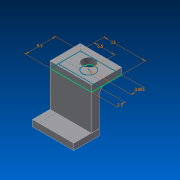
# Autodesk Inventor part: ethernet bracket support
Saved by Autodesk Inventor 2015 (Build 190159000, 159)
## iProperties
Created: 2017-03-16
Part Number: ethernet bracket support
Material: Generic
Document SubType Name: Modeling
Designer: ZigZagJoe
Density: 1 g/cm^3
Appearance: Default
Author: ZigZagJoe
Autodesk Inventor part; units mm, degrees
ref_plane "YZ Plane" through (0, 0, 0) normal (1, 0, 0) x (0, 1, 0)
ref_plane "XZ Plane" through (0, 0, 0) normal (0, 1, 0) x (-1, 0, 0)
ref_plane "XY Plane" through (0, 0, 0) normal (0, 0, 1) x (1, 0, 0)
sketch "Sketch1" plane through (0, 0, 0) normal (0, 0, 1) x (1, 0, 0)
  line L0 (-5.976, 1.765) -> (7.024, 1.765)
  line L1 (7.024, 1.765) -> (7.024, -7.735)
  line L2 (7.024, -7.735) -> (-5.976, -7.735)
  line L3 (-5.976, -7.735) -> (-5.976, 1.765)
  line L4 (-5.976, -7.735) -> (7.024, -7.735)
  line L5 (7.024, -7.735) -> (7.024, -5.235)
  line L6 (7.024, -5.235) -> (-5.976, -5.235)
  line L7 (-5.976, -5.235) -> (-5.976, -7.735)
  circle A0 centre (0.524, -2.0964) radius 2
  point P0 (0, 0)
  dimension "d0" = 9.5
  dimension "d1" = 13
  dimension "d2" = 2.5
  dimension "d3" = 4
  dimension "d4" = 6.5
  dimension "d5" = 3.8614
  constraints: 16 end point, 4 parallel, 2 horizontal, 2 perpendicular, 1 centre point, 1 point on line
  measures "d0" distance of L2.end L0.start
  measures "d1" distance of L0.start L0.end
  measures "d2" distance between parallel lines of L2 L6
  measures "d3" diameter of A0
  measures "d4" distance from line of L3 A0.centre
  measures "d5" distance from line of L0 A0.centre
extrude "Extrusion1" add sketch "Sketch1" along normal blind 2
extrude "Extrusion2" add sketch "Sketch1" against normal blind 11.2 contours L6 L1 L2 L3
sketch "Sketch2" plane through (0, 0, -11.2) normal (0, 0, -1) x (-1, 0, 0)
  line L0 (-6.988, -5.235) -> (5.976, -5.235)
  line L1 (5.976, -5.235) -> (5.976, -13.235)
  line L2 (5.976, -13.235) -> (-6.988, -13.235)
  line L3 (-6.988, -13.235) -> (-6.988, -5.235)
  line L4 (5.976, -7.735) -> (5.976, -5.235) projected
  line L5 (5.976, -5.235) -> (-7.024, -5.235) projected
  point P0 (0, 0)
  dimension "d10" = 0
  dimension "d11" = 8
  dimension "d12" = 0
  constraints: 8 end point, 2 parallel, 1 horizontal, 1 perpendicular
  measures "d10" distance between parallel lines of L1 L4
  measures "d11" distance of L2.end L0.start
  measures "d12" distance between parallel lines of L5 L0
extrude "Extrusion3" add sketch "Sketch2" along normal blind 2
fillet "Fillet1" radius 2 1 edges at (0.524, -5.235, 0)
body "Solid1"
